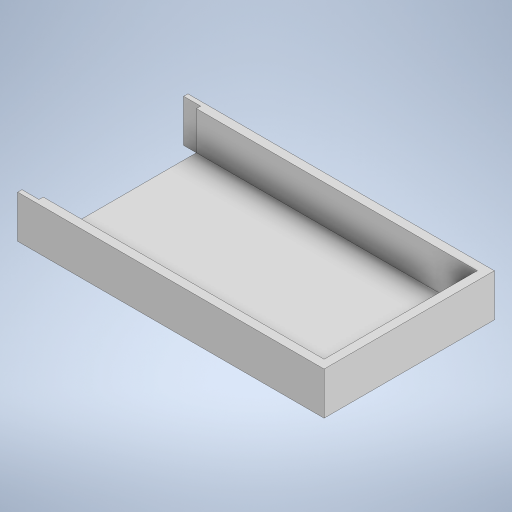
# Autodesk Inventor part: Schublade Teil B
Saved by Autodesk Inventor 2023 (Build 270158000, 158)
## iProperties
Created: 2023-08-28
Part Number: Schublade Teil B
Material: Generisch
Document SubType Name: Modeling
Designer: elueders
Density: 1 g/cm^3
Appearance: Vorgabe
Author: elueders
Autodesk Inventor part; units mm, degrees
ref_plane "YZ Plane" through (0, 0, 0) normal (1, 0, 0) x (0, 1, 0)
ref_plane "XZ Plane" through (0, 0, 0) normal (0, 1, 0) x (-1, 0, 0)
ref_plane "XY Plane" through (0, 0, 0) normal (0, 0, 1) x (1, 0, 0)
sketch "Skizze1" plane through (0, 0, 0) normal (0, 1, 0) x (-1, 0, 0)
  line L0 (0, 0) -> (180, 0)
  line L1 (180, -100) -> (0, -100)
  line L2 (0, -100) -> (0, 0)
  line L3 (5, -95) -> (5, -5)
  line L4 (5, -5) -> (170, -5)
  line L5 (5, -95) -> (170, -95)
  line L6 (170, -95) -> (170, -97.5)
  line L7 (170, -97.5) -> (180, -97.5)
  line L8 (170, -5) -> (170, -2.5)
  line L9 (170, -2.5) -> (180, -2.5)
  line L10 (180, 0) -> (180, -2.5)
  line L11 (180, -100) -> (180, -97.5)
  dimension "d0" = 180
  dimension "d1" = 100
  dimension "d2" = 90
  dimension "d3" = 165
  constraints: 24 end point, 3 horizontal, 2 equal length, 2 vertical
  measures "d0" distance of L1.start L1.end
  measures "d1" distance of L0.end L1.start
  measures "d2" distance of L3.start L3.end
  measures "d3" distance of L3.start L5.end
extrude "Extrusion1" add sketch "Skizze1" along normal blind 25
sketch "Skizze2" plane through (-5, 0, -95) normal (-1, 0, 0) x (0, 0, 1)
  line L0 (90, 0) -> (90, 25) projected
  line L1 (0, 0) -> (90, 0) projected
  line L2 (90, 0) -> (90, 25) projected
  line L3 (0, 25) -> (90, 25) projected
  line L4 (0, 0) -> (0, 25) projected
  line L5 (0, 0) -> (90, 0)
  line L6 (90, 0) -> (90, 2.5)
  line L7 (90, 2.5) -> (0, 2.5)
  line L8 (0, 2.5) -> (0, 0)
  point P0 (95, 0)
  dimension "d6" = 90
  dimension "d7" = 2.5
  constraints: 8 end point, 2 parallel, 1 horizontal, 1 perpendicular
  measures "d6" distance of L7.end L6.end
  measures "d7" distance of L6.end L5.end
extrude "Extrusion2" add sketch "Skizze2" along normal blind 165 contours L1 L4 L7 L0
